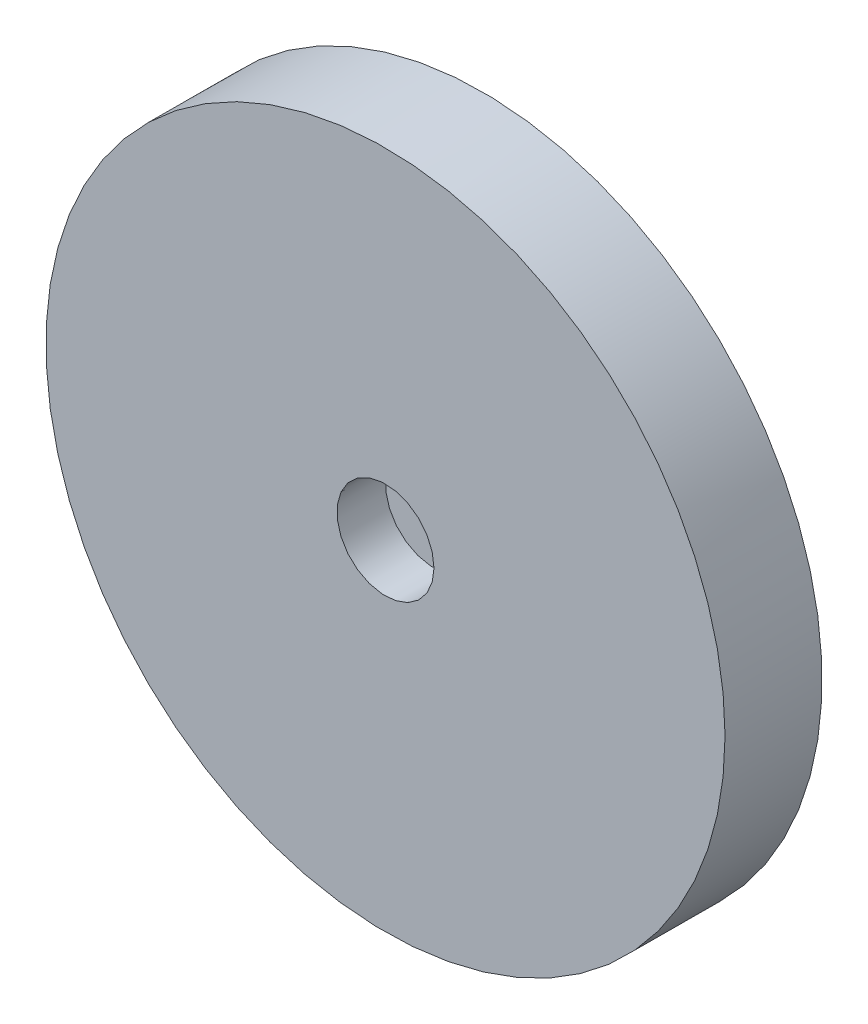
# Autodesk Inventor part: крышка
Saved by Autodesk Inventor 2024.2 (Build 282272000, 272)
## iProperties
Created: 2025-12-24
Part Number: крышка
Material: Типовые
Document SubType Name: Modeling
Designer: katya_notebook
Density: 1 g/cm^3
Appearance: По умолчанию
Author: katya_notebook
Autodesk Inventor part; units mm, degrees
ref_plane "YZ Plane" through (0, 0, 0) normal (1, 0, 0) x (0, 1, 0)
ref_plane "XZ Plane" through (0, 0, 0) normal (0, 1, 0) x (-1, 0, 0)
ref_plane "РабПлоскость1" through (1955.2464, 20.5, -10) normal (0, 0, 1) x (1, 0, 0)
sketch "Эскиз1" plane through (1955.2464, 20.5, -10) normal (0, 0, 1) x (1, 0, 0)
  circle A0 centre (0, 0) radius 14
  circle A1 centre (0, 0) radius 12.25
  point P0 (-1955.2464, -20.5)
  dimension "d0" = 28
  dimension "d1" = 24.5
  constraints: 2 centre point, 1 coincident
  measures "d0" diameter of A0
  measures "d1" diameter of A1
ref_plane "РабПлоскость2" through (1941.2464, 6.5, -14) normal (0, 0, 1) x (1, 0, 0)
extrude "Выдавливание1" add sketch "Эскиз1" against normal up to surface (4 mm away)
sketch "Эскиз2" plane through (1955.2464, 20.5, -10) normal (0, 0, 1) x (1, 0, 0)
  circle A0 centre (0, 0) radius 14
  point P0 (-1955.2464, -20.5)
  constraints: 1 centre point
extrude "Выдавливание2" add sketch "Эскиз2" against normal blind 2.5
sketch "Эскиз3" plane through (1955.2464, 20.5, -12.5) normal (0, 0, -1) x (-1, 0, 0)
  circle A0 centre (0, 0) radius 2
  point P0 (1955.2464, -20.5)
  dimension "d6" = 4
  constraints: 1 centre point
  measures "d6" diameter of A0
sketch "Эскиз4" plane through (1955.2464, 20.5, -10) normal (0, 0, 1) x (1, 0, 0)
  circle A0 centre (0, 0) radius 2
  point P0 (-1955.2464, -20.5)
  dimension "d9" = 4
  constraints: 1 centre point
  measures "d9" diameter of A0
extrude "Выдавливание4" cut sketch "Эскиз4" against normal blind 2
